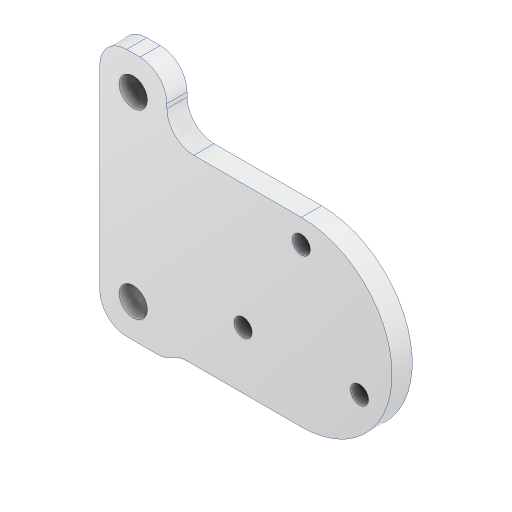
# Autodesk Inventor part: finger2
Saved by Autodesk Inventor 2024.3 (Build 283343000, 343)
## iProperties
Created: 2024-10-15
Part Number: finger2
Material: アルミニウム 6061
Document SubType Name: Modeling
Designer: haya
Density: 2.7 g/cm^3
Appearance: アルミニウム - フラット
Mass: 7.08365 g
Surface Area: 22.7219 cm^2
Volume: 2.62357 cm^3
Author: haya
Autodesk Inventor part; units mm, degrees
ref_plane "YZ Plane" through (0, 0, 0) normal (1, 0, 0) x (0, 1, 0)
ref_plane "XZ Plane" through (0, 0, 0) normal (0, 1, 0) x (-1, 0, 0)
ref_plane "XY Plane" through (0, 0, 0) normal (0, 0, 1) x (1, 0, 0)
sketch "スケッチ1" plane through (0, 0, 0) normal (0, 0, 1) x (1, 0, 0)
  circle A0 centre (0, 0) radius 13.5
  dimension "d0" = 27
  constraints: 1 centre point, 1 coincident
  measures "d0" diameter of A0
extrude "押し出し1" add sketch "スケッチ1" along normal blind 3
sketch "スケッチ2" plane through (0, 0, 3) normal (0, 0, 1) x (1, 0, 0)
  point P0 (0, 0)
  point P1 (0, 10)
  point P2 (-8.6603, -5)
  point P3 (8.6603, -5)
  dimension "d3" = 10
  dimension "d6" = 360
  constraints: 4 other
  measures "d3" distance of point (0, 10) point (0, 0)
hole "穴1" at (0, 10, 3) at (-8.6603, -5, 3) at (8.6603, -5, 3) direction (0, 0, -1) diameter 2.7 depth 3 tip angle 118
sketch "スケッチ3" plane through (0, 0, 0) normal (0, 0, -1) x (-1, 0, 0)
  circle A0 centre (0, 0) radius 13.5 projected
  line L0 (0, -13.5) -> (30, -13.5)
  line L1 (30, -13.5) -> (30, 13.5)
  line L2 (30, 13.5) -> (0, 13.5)
  line L3 (0, 13.5) -> (0, -13.5)
  line L4 (0, 0) -> (30, 0) construction
  line L5 (30, 13.5) -> (20, 13.5)
  line L6 (20, 13.5) -> (20, 22.15)
  line L7 (20, 22.15) -> (30, 22.15)
  line L8 (30, 22.15) -> (30, 13.5)
  line L9 (30, -13.5) -> (20, -13.5)
  line L10 (20, -13.5) -> (20, -14.85)
  line L11 (20, -14.85) -> (30, -14.85)
  line L12 (30, -14.85) -> (30, -13.5)
  dimension "d15" = 27
  dimension "d16" = 30
  dimension "d18" = 10
  dimension "d32" = 10
  dimension "d33" = 1.35
  dimension "d34" = 37
  constraints: 26 end point, 6 parallel, 3 horizontal, 3 perpendicular, 1 midpoint, 3 other
  measures "d15" distance of L0.end L1.end
  measures "d16" distance of L0.start L0.end
  measures "d18" distance of L6.end L7.end
  measures "d32" distance of L10.end L11.end
  measures "d33" distance between parallel lines of L0 L11
  measures "d34" distance between parallel lines of L11 L7
extrude "押し出し2" add sketch "スケッチ3" against normal up to surface (3 mm away) contours A0 L2 L1 L0 | L6 L7 L8 L2 | L0 L12 L11 L10
sketch "スケッチ4" plane through (0, 0, 0) normal (0, 0, -1) x (-1, 0, 0)
  line L0 (0, -13.5) -> (20, -13.5) projected
  line L1 (25, -13.5) -> (25, 22.15) construction
  line L2 (30, 22.15) -> (20, 22.15) projected
  line L3 (20, -14.85) -> (30, -14.85) projected
  line L4 (30, -14.85) -> (30, 22.15) projected
  point P0 (0, 0)
  point P1 (25, -9.85)
  point P2 (25, 17.15)
  dimension "d23" = 27
  dimension "d35" = 5
  dimension "d37" = 5
  constraints: 3 point on line, 2 end point, 1 midpoint, 1 vertical
  measures "d23" distance of point (25, 17.15) point (25, -9.85)
  measures "d35" distance from line of L3 point (25, -9.85)
  measures "d37" distance from line of point (25, -9.85) L4
hole "穴2" at (-25, -9.85, 0) at (-25, 17.15, 0) direction (0, 0, 1) diameter 4.2 depth 3 tip angle 118
fillet "フィレット1" radius 4 6 edges at (-20, 13.5, 1.5) (-20, 22.15, 1.5) (-30, 22.15, 1.5) (-30, -14.85, 1.5) (-20, -14.85, 1.5) (-20, -13.5, 1.5)
